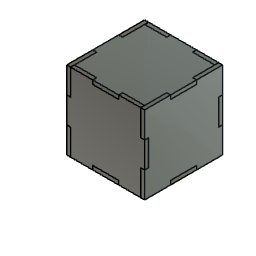
box (Autodesk Fusion 360 design; units mm, degrees)
Autodesk Fusion 360 part; units mm, degrees
sketch "bottom sketch" plane through (0, 0, 0) normal (0, 0, 1) x (1, 0, 0)
  line L0 (0, 0) -> (60, 0)
  line L1 (60, 0) -> (60, 60)
  line L2 (60, 60) -> (0, 60)
  line L3 (0, 60) -> (0, 0)
  dimension "d8" = 60
  dimension "d9" = 60
  constraint horizontal L0
  constraint vertical L1
  constraint horizontal L2
  constraint vertical L3
  constraint coincident L0.start L3.end
  measures "d8" distance of L0.start L0.end
  measures "d9" distance of L0.start L2.end
extrude "Extrude1" add sketch "bottom sketch" along normal blind 3 makes body 1
sketch "front sketch" plane through (0, 0, 0) normal (0, -1, 0) x (1, 0, 0)
  line L0 (0, 0) -> (60, 0)
  line L1 (60, 0) -> (60, 3)
  line L2 (60, 3) -> (0, 3)
  line L3 (0, 3) -> (0, 0)
  line L4 (0, 0) -> (60, 0)
  line L5 (60, 0) -> (60, 60)
  line L6 (60, 60) -> (0, 60)
  line L7 (0, 60) -> (0, 0)
  line L8 (0, 0) -> (20, 0)
  line L9 (20, 0) -> (20, 3)
  line L10 (20, 3) -> (0, 3)
  line L11 (0, 3) -> (0, 0)
  line L12 (20, 0) -> (40, 0)
  line L13 (40, 0) -> (40, 3)
  line L14 (40, 3) -> (20, 3)
  line L15 (20, 3) -> (20, 0)
  dimension "d12" = 60
  dimension "d13" = 60
  dimension "d14" = 20
  dimension "d15" = 20
  constraint horizontal L4
  constraint vertical L5
  constraint horizontal L6
  constraint vertical L7
  constraint coincident L0.start L3.end
  constraint horizontal L8
  constraint vertical L9
  constraint horizontal L10
  constraint vertical L11
  constraint coincident L2 L9.end
  constraint horizontal L12
  constraint vertical L13
  constraint horizontal L14
  constraint vertical L15
  constraint coincident L2 L13.end
  measures "d12" distance of L0.start L0.end
  measures "d13" distance of L0.start L6.end
  measures "d14" distance of L0.start L8.end
  measures "d15" distance of L8.end L12.end
extrude "Extrude2" add sketch "front sketch" against normal blind 3 separate body contours L0 L2 L3 L4 L7 L8 L9 L10 L11 L15 | L2 L5 L6 L7 L10 L14 | L0 L1 L2 L4 L5 L13 makes body 2
combine "Combine1" operation cut target body 1 tool bodies 2 keep tools
ref_plane "WorkPlane1" through (30, 30, 1.5) normal (0, 1, 0) x (-1, 0, 0)
mirror "Mirror1" about plane through (30, 30, 1.5) normal (0, 1, 0) of bodies 2 makes body 3
combine "Combine2" operation cut target body 1 tool bodies 3 keep tools
sketch "left sketch" plane through (0, 0, 0) normal (1, 0, 0) x (0, 1, 0)
  line L0 (0, 0) -> (60, 0)
  line L1 (60, 0) -> (60, 60)
  line L2 (60, 60) -> (0, 60)
  line L3 (0, 60) -> (0, 0)
  line L4 (0, 0) -> (20, 0)
  line L5 (20, 0) -> (20, 3)
  line L6 (20, 3) -> (0, 3)
  line L7 (0, 3) -> (0, 0)
  line L8 (57, 3) -> (3, 3)
  line L9 (20, 0) -> (40, 0)
  line L10 (40, 0) -> (40, 3)
  line L11 (40, 3) -> (20, 3)
  line L12 (20, 3) -> (20, 0)
  line L13 (0, 0) -> (3, 0)
  line L14 (3, 0) -> (3, 20)
  line L15 (3, 20) -> (0, 20)
  line L16 (0, 20) -> (0, 0)
  line L17 (0, 20) -> (3, 20)
  line L18 (3, 20) -> (3, 40)
  line L19 (3, 40) -> (0, 40)
  line L20 (0, 40) -> (0, 20)
  line L21 (60, 0) -> (57, 0)
  line L22 (57, 0) -> (57, 20)
  line L23 (57, 20) -> (60, 20)
  line L24 (60, 20) -> (60, 0)
  line L25 (60, 20) -> (57, 20)
  line L26 (57, 20) -> (57, 40)
  line L27 (57, 40) -> (60, 40)
  line L28 (60, 40) -> (60, 20)
  dimension "d19" = 60
  dimension "d20" = 60
  dimension "d21" = 20
  dimension "d22" = 20
  dimension "d23" = 3
  dimension "d24" = 20
  dimension "d25" = 3
  dimension "d26" = 20
  dimension "d27" = 3
  dimension "d28" = 20
  dimension "d29" = 3
  dimension "d30" = 20
  constraint horizontal L0
  constraint vertical L1
  constraint horizontal L2
  constraint vertical L3
  constraint coincident L0.start L3.end
  constraint horizontal L4
  constraint vertical L5
  constraint horizontal L6
  constraint vertical L7
  constraint coincident L5.end L8
  constraint horizontal L9
  constraint vertical L10
  constraint horizontal L11
  constraint vertical L12
  constraint coincident L8 L10.end
  constraint horizontal L13
  constraint vertical L14
  constraint horizontal L15
  constraint vertical L16
  constraint horizontal L17
  constraint vertical L18
  constraint horizontal L19
  constraint vertical L20
  constraint horizontal L21
  constraint vertical L22
  constraint horizontal L23
  constraint vertical L24
  constraint horizontal L25
  constraint vertical L26
  constraint horizontal L27
  constraint vertical L28
  measures "d19" distance of L0.start L0.end
  measures "d20" distance of L0.start L2.end
  measures "d21" distance of L0.start L4.end
  measures "d22" distance of L4.end L9.end
  measures "d23" distance of L0.start L13.end
  measures "d24" distance of L0.start L15.end
  measures "d25" distance of L15.end L14.end
  measures "d26" distance of L15.end L19.end
  measures "d27" distance of L0.end L21.end
  measures "d28" distance of L0.end L23.end
  measures "d29" distance of L23.end L22.end
  measures "d30" distance of L23.end L27.end
extrude "Extrude3" add sketch "left sketch" along normal blind 3 separate body contours L0 L3 L4 L6 L7 L13 L14 L16 | L0 L4 L5 L6 L8 L12 L14 | L3 L6 L14 L15 L16 L17 | L1 L2 L3 L6 L8 L11 L14 L18 L19 L22 L26 L27 | L0 L8 L10 L22 | L0 L1 L21 L22 L23 L24 L25 makes body 4
combine "Combine3" operation cut target body 1 tool bodies 4 keep tools
ref_plane "WorkPlane2" through (30, 30, 1.5) normal (-1, 0, 0) x (0, -1, 0)
mirror "Mirror2" about plane through (30, 30, 1.5) normal (-1, 0, 0) of bodies 4 makes body 5
combine "Combine4" operation cut target body 1 tool bodies 5 keep tools
combine "Combine5" operation cut target body 3 tool bodies 5 4 keep tools
combine "Combine6" operation cut target body 2 tool bodies 5 4 keep tools
ref_plane "WorkPlane3" through (30, 30, 30) normal (0, 0, -1) x (-1, 0, 0)
mirror "Mirror3" about plane through (30, 30, 30) normal (0, 0, -1) of bodies 1 makes body 6
combine "Combine7" operation cut target body 2 tool bodies 6 keep tools
combine "Combine8" operation cut target body 5 tool bodies 6 keep tools
combine "Combine9" operation cut target body 3 tool bodies 6 keep tools
combine "Combine10" operation cut target body 4 tool bodies 6 keep tools
sketch "top-dxf" plane through (0, 0, 60) normal (0, 0, 1) x (-1, 0, 0)
  line L0 (-57, -40) -> (-57, -57)
  line L1 (-57, -57) -> (-40, -57)
  line L2 (-40, -57) -> (-40, -60)
  line L3 (-40, -60) -> (-20, -60)
  line L4 (-20, -60) -> (-20, -57)
  line L5 (-20, -57) -> (-3, -57)
  line L6 (-3, -57) -> (-3, -40)
  line L7 (-3, -40) -> (0, -40)
  line L8 (0, -40) -> (0, -20)
  line L9 (0, -20) -> (-3, -20)
  line L10 (-3, -20) -> (-3, -3)
  line L11 (-3, -3) -> (-20, -3)
  line L12 (-20, -3) -> (-20, 0)
  line L13 (-20, 0) -> (-40, 0)
  line L14 (-40, 0) -> (-40, -3)
  line L15 (-40, -3) -> (-57, -3)
  line L16 (-57, -3) -> (-57, -20)
  line L17 (-57, -20) -> (-60, -20)
  line L18 (-60, -20) -> (-60, -40)
  line L19 (-60, -40) -> (-57, -40)
sketch "right-dxf" plane through (60, 0, 0) normal (1, 0, 0) x (0, 1, 0)
  line L0 (20, 57) -> (20, 60)
  line L1 (20, 60) -> (0, 60)
  line L2 (0, 60) -> (0, 40)
  line L3 (0, 40) -> (3, 40)
  line L4 (3, 40) -> (3, 20)
  line L5 (3, 20) -> (0, 20)
  line L6 (0, 20) -> (0, 0)
  line L7 (0, 0) -> (20, 0)
  line L8 (20, 0) -> (20, 3)
  line L9 (20, 3) -> (40, 3)
  line L10 (40, 3) -> (40, 0)
  line L11 (40, 0) -> (60, 0)
  line L12 (60, 0) -> (60, 20)
  line L13 (60, 20) -> (57, 20)
  line L14 (57, 20) -> (57, 40)
  line L15 (57, 40) -> (60, 40)
  line L16 (60, 40) -> (60, 60)
  line L17 (60, 60) -> (40, 60)
  line L18 (40, 60) -> (40, 57)
  line L19 (40, 57) -> (20, 57)
sketch "back-dxf" plane through (0, 60, 0) normal (0, 1, 0) x (-1, 0, 0)
  line L0 (-40, 57) -> (-40, 60)
  line L1 (-40, 60) -> (-57, 60)
  line L2 (-57, 60) -> (-57, 40)
  line L3 (-57, 40) -> (-60, 40)
  line L4 (-60, 40) -> (-60, 20)
  line L5 (-60, 20) -> (-57, 20)
  line L6 (-57, 20) -> (-57, 0)
  line L7 (-57, 0) -> (-40, 0)
  line L8 (-40, 0) -> (-40, 3)
  line L9 (-40, 3) -> (-20, 3)
  line L10 (-20, 3) -> (-20, 0)
  line L11 (-20, 0) -> (-3, 0)
  line L12 (-3, 0) -> (-3, 20)
  line L13 (-3, 20) -> (0, 20)
  line L14 (0, 20) -> (0, 40)
  line L15 (0, 40) -> (-3, 40)
  line L16 (-3, 40) -> (-3, 60)
  line L17 (-3, 60) -> (-20, 60)
  line L18 (-20, 60) -> (-20, 57)
  line L19 (-20, 57) -> (-40, 57)
equation "length = 60 mm" comment "cube length"
equation "width = 60 mm" comment "cube width"
equation "height = 60 mm" comment "cube height"
equation "thickness = 3 mm" comment "thickness"
equation "fingerL = length / 3" comment "finger on length"
equation "fingerW = width / 3" comment "finger on width"
equation "fingerH = height / 3" comment "finger on height"
equation "d8 = length"
equation "d9 = width"
equation "d10 = thickness"
equation "d12 = length"
equation "d13 = height"
equation "d14 = fingerL"
equation "d15 = fingerL"
equation "d16 = -thickness"
equation "d19 = width"
equation "d20 = height"
equation "d21 = fingerW"
equation "d22 = fingerW"
equation "d23 = thickness"
equation "d24 = fingerH"
equation "d25 = thickness"
equation "d26 = fingerH"
equation "d27 = thickness"
equation "d28 = fingerH"
equation "d29 = thickness"
equation "d30 = fingerH"
equation "d31 = thickness"
named bodies: "bottom", "front", "back", "left", "right", "top"
